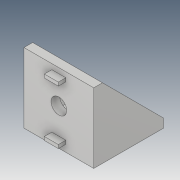
# Autodesk Inventor part: Gusset_4040_8
Saved by Autodesk Inventor 2018 (Build 220112000, 112)
## iProperties
Created: 2017-10-23
Part Number: Gusset_4040_8
Material: Aluminum
Document SubType Name: Modeling
Designer: NicK Foo
Density: 2.7 g/cm^3
Appearance: Satin
Author: NicK Foo
Autodesk Inventor part; units mm, degrees
ref_plane "YZ Plane" through (0, 0, 0) normal (1, 0, 0) x (0, 1, 0)
ref_plane "XZ Plane" through (0, 0, 0) normal (0, 1, 0) x (-1, 0, 0)
ref_plane "XY Plane" through (0, 0, 0) normal (0, 0, 1) x (1, 0, 0)
sketch "Sketch1" plane through (0, 0, 0) normal (1, 0, 0) x (0, 1, 0)
  line L0 (0, 0) -> (40, 0)
  line L1 (40, 0) -> (40, -5)
  line L2 (40, -40) -> (5, -40) construction
  line L3 (0, -40) -> (0, 0)
  line L4 (40, 0) -> (40, -5)
  line L5 (40, -5) -> (5, -40)
  line L6 (0, -40) -> (5, -40)
  line L7 (40, -5) -> (5, -5)
  line L8 (5, -5) -> (5, -40)
  line L9 (40, -5) -> (40, -40) construction
  line L10 (5, -40) -> (0, -40)
  line L11 (37, 0) -> (35, 0)
  line L12 (35, 0) -> (35, 4.3)
  line L13 (35, 4.3) -> (37, 4.3)
  line L14 (37, 4.3) -> (37, 0)
  line L15 (6, 0) -> (4, 0)
  line L16 (4, 0) -> (4, 4.3)
  line L17 (4, 4.3) -> (6, 4.3)
  line L18 (6, 4.3) -> (6, 0)
  point P0 (5, 0)
  dimension "d0" = 40
  dimension "d1" = 5
  dimension "d2" = 2
  dimension "d3" = 4.3
  dimension "d4" = 4
  dimension "d5" = 3
  constraints: 38 end point, 8 parallel, 7 perpendicular, 5 point on line, 3 collinear, 3 equal length, 1 horizontal, 1 midpoint
  measures "d0" distance of L0.start L0.end
  measures "d1" distance of L0.end L1.end
  measures "d2" distance of L11.start L11.end
  measures "d3" distance of L13.end L11.start
  measures "d4" distance between parallel lines of L3 L16
  measures "d5" distance between parallel lines of L1 L14
extrude "Extrusion1" add sketch "Sketch1" along normal mid plane 40 contours L0 L1 L7 L8 L6 L3 | L8 L7 L5
extrude "Extrusion2" cut sketch "Sketch1" along normal mid plane 30 contours L8 L7 L5
extrude "Extrusion3" add sketch "Sketch1" along normal mid plane 8 contours L16 L17 L18 L0 | L12 L13 L14 L0
sketch "Sketch2" plane through (15, 5, -5) normal (0, 1, 0) x (-1, 0, 0)
  line L0 (15, -10) -> (15, -25) construction
  line L1 (10.5, -10) -> (10.5, -25)
  line L2 (19.5, -25) -> (19.5, -10)
  arc A0 (19.5, -10) -> (10.5, -10) centre (15, -10) ccw
  arc A1 (10.5, -25) -> (19.5, -25) centre (15, -25) ccw
  line L3 (30, 0) -> (0, 0) projected
  point P0 (15, 5)
  point P1 (15, -17.5)
  point P2 (15, 0)
  dimension "d12" = 15
  dimension "d13" = 9
  dimension "d14" = 10
  constraints: 8 end point, 4 point on circle, 4 tangent, 2 centre point, 2 midpoint, 1 parallel, 1 point on line, 1 vertical
  measures "d12" distance of L0.start L0.end
  measures "d13" diameter of A1
  measures "d14" distance from line of L3 L0.start
extrude "Extrusion4" cut sketch "Sketch2" against normal through all
sketch "Sketch3" plane through (-15, 5, -5) normal (0, 0, -1) x (1, 0, 0)
  line L0 (-5, 5) -> (35, 5) projected
  circle A0 centre (15, -16) radius 4.5
  line L1 (0, -35) -> (30, -35) projected
  line L2 (15, -16) -> (15, -35) construction
  point P0 (15, 5)
  dimension "d18" = 9
  dimension "d21" = 19
  constraints: 2 end point, 1 centre point, 1 midpoint, 1 perpendicular
  measures "d18" diameter of A0
  measures "d21" distance from line of L1 L2.start
extrude "Extrusion5" cut sketch "Sketch3" against normal through all
body "Solid1"
